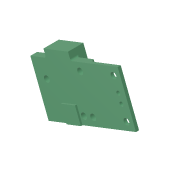
# Autodesk Inventor part: VWheelArmThickRIghtThinSwitchMount
Saved by Autodesk Inventor 2018 (Build 220112000, 112)
## iProperties
Created: 2018-12-14
Part Number: VWheelArmThickRIghtThinSwitchMount
Material: Generic
Document SubType Name: Modeling
Designer: ball
Density: 1 g/cm^3
Appearance: Default
Author: ball
Autodesk Inventor part; units mm, degrees
ref_plane "YZ Plane" through (0, 0, 0) normal (1, 0, 0) x (0, 1, 0)
ref_plane "XZ Plane" through (0, 0, 0) normal (0, 1, 0) x (-1, 0, 0)
ref_plane "XY Plane" through (0, 0, 0) normal (0, 0, 1) x (1, 0, 0)
sketch "Sketch1" plane through (0, 0, 0) normal (0, 0, 1) x (1, 0, 0)
  circle A0 centre (50.1681, 27.2834) radius 1.778 construction
  circle A1 centre (25.0574, 17.5233) radius 1.778 construction
  circle A2 centre (34.8176, -7.5874) radius 1.778 construction
  circle A3 centre (59.9282, 2.1728) radius 1.778 construction
  circle A4 centre (0, 0) radius 3.5 construction
  circle A5 centre (44.7061, 31.1467) radius 1.778 construction
  circle A6 centre (58.509, -4.3651) radius 1.778 construction
  circle A7 centre (26.4767, 24.0612) radius 1.778 construction
  circle A8 centre (40.2796, -11.4506) radius 1.778 construction
  line L0 (44.7061, 31.1467) -> (26.4767, 24.0612) construction
  line L1 (58.509, -4.3651) -> (40.2796, -11.4506) construction
  line L2 (168.5413, -268.1733) -> (30.5122, 86.945) construction
  circle A9 centre (-14.8554, 15.0432) radius 1.778 construction
  circle A10 centre (1.8062, -27.8234) radius 1.778 construction
  line L3 (67.1502, -1.0064) -> (1.3271, -26.5908)
  line L4 (53.3473, 34.5054) -> (-12.4758, 8.921)
  line L5 (-12.4758, 8.921) -> (1.3271, -26.5908)
  circle A11 centre (50.1681, 27.2834) radius 2.2479
  circle A12 centre (59.9282, 2.1728) radius 2.2479
  circle A13 centre (34.8176, -7.5874) radius 2.2479
  circle A14 centre (25.0574, 17.5233) radius 2.2479
  circle A15 centre (0, 0) radius 2.2479
  line L6 (53.3473, 34.5054) -> (67.1502, -1.0064)
  circle A16 centre (27.9489, -10.2481) radius 2.2479
  point P0 (51.2166, 33.6772)
  dimension "d0" = 4.4958
  dimension "d1" = 4.4958
  dimension "d2" = 4.4958
  dimension "d3" = 4.4958
  dimension "d4" = 4.4958
  dimension "d28" = 4.4958
  dimension "d29" = 7.366
  dimension "d30" = 5.5796
  dimension "d31" = 5.588
  constraints: 17 centre point, 14 end point, 5 coincident, 4 point on line, 28 other
  measures "d0" diameter of A11
  measures "d1" diameter of A12
  measures "d2" diameter of A13
  measures "d3" diameter of A14
  measures "d4" diameter of A15
  measures "d28" diameter of A16
  measures "d29" distance of A2.centre A16.centre
  measures "d30" distance from line of L3 A13.centre
  measures "d31" distance from line of L3 A16.centre
extrude "Extrusion1" add sketch "Sketch1" along normal blind 2.286 contours L3 L5 L4 L6 | A16
sketch "Sketch2" plane through (0, 0, 0) normal (0, 0, -1) x (-1, 0, 0)
  line L0 (12.4758, 8.921) -> (-1.3271, -26.5908) projected
  line L1 (12.4758, 8.921) -> (-1.3271, -26.5908)
  line L2 (-1.3271, -26.5908) -> (-43.9413, -10.0274)
  line L3 (-43.9413, -10.0274) -> (-30.1384, 25.4845)
  line L4 (-30.1384, 25.4845) -> (12.4758, 8.921)
  circle A0 centre (0, 0) radius 2.2479 projected
  circle A1 centre (-34.8176, -7.5874) radius 2.2479 projected
  circle A2 centre (-25.0574, 17.5233) radius 2.2479 projected
  dimension "d7" = 45.72
  constraints: 8 end point, 3 equal length, 1 perpendicular
  measures "d7" distance of L3.end L0.start
extrude "Extrusion2" add sketch "Sketch2" along normal blind 2.794
sketch "Sketch3" plane through (0, 0, -2.794) normal (0, 0, -1) x (-1, 0, 0)
  line L0 (-19.647, 16.2289) -> (-16.4172, 24.5387) construction
  line L1 (2.3869, 18.0201) -> (-1.1099, 9.0238) construction
  circle A0 centre (-5.0584, 13.1678) radius 1.1938 construction
  circle A1 centre (-13.9363, 16.6185) radius 1.1938 construction
  line L2 (-6.3321, 22.0903) -> (2.0251, 18.842) construction
  line L3 (-1.1099, 9.0238) -> (-19.647, 16.2289)
  line L4 (-19.647, 16.2289) -> (-15.9203, 25.8171)
  line L5 (-15.9203, 25.8171) -> (2.6169, 18.612)
  line L6 (2.6169, 18.612) -> (-1.1099, 9.0238)
  circle A2 centre (-5.0584, 13.1678) radius 1.1938
  circle A3 centre (-13.9363, 16.6185) radius 1.1938
  point P0 (0, 0)
  constraints: 14 end point, 4 centre point, 2 coincident, 2 concentric, 2 parallel, 1 perpendicular, 13 other
ref_plane "Work Plane1" through (-2.6408, 8.9775, -9.2647) normal (0, 0, 1) x (0.9320689, 0.3622811, 0)
extrude "Extrusion3" add sketch "Sketch3" along normal up to surface (6.4707 mm away)
sketch "Sketch4" plane through (0, 0, -2.794) normal (0, 0, 1) x (1, 0, 0)
  line L0 (-0.6385, 13.5219) -> (17.8987, 20.7271) projected
  line L1 (17.8987, 20.7271) -> (-0.6385, 13.5219)
  line L2 (-0.6385, 13.5219) -> (-2.6169, 18.612)
  line L3 (-2.6169, 18.612) -> (15.9203, 25.8171)
  line L4 (15.9203, 25.8171) -> (17.8987, 20.7271)
  point P0 (0, 0)
  constraints: 8 end point, 3 equal length, 1 perpendicular
extrude "Extrusion4" add sketch "Sketch4" along normal up to surface (5.08 mm away)
fillet "Fillet1" radius 3.175 1 edges at (37.0399, 7.7286, 0)
sketch "Sketch5" plane through (0, 0, 0) normal (0, 0, -1) x (-1, 0, 0)
  circle A0 centre (-50.1681, 27.2834) radius 2.2479 construction
  circle A1 centre (-59.9282, 2.1728) radius 2.2479 construction
  line L0 (-50.1681, 27.2834) -> (-59.9282, 2.1728) construction
  circle A2 centre (-53.8949, 17.6952) radius 1.524
  circle A3 centre (-56.1954, 11.7766) radius 1.524
  point P0 (0, 0)
  dimension "d15" = 3.048
  dimension "d16" = 3.048
  dimension "d17" = 6.35
  dimension "d18" = 10.287
  constraints: 2 centre point, 2 end point, 2 point on line
  measures "d15" diameter of A2
  measures "d16" diameter of A3
  measures "d17" distance of A3.centre A2.centre
  measures "d18" distance of A2.centre L0.start
extrude "Extrusion5" cut sketch "Sketch5" along normal through all both and the other way through all
fillet "Fillet2" radius 1.27 3 edges at (10.3785, 12.6263, -2.794) (18.7729, 18.478, -2.794) (0.2357, 11.2729, -2.794)
fillet "Fillet3" radius 1.27 4 edges at (17.8987, 20.7271, -3.429) (17.8987, 20.7271, -0.254) (-0.6385, 13.5219, -3.429) (-0.6385, 13.5219, -0.254)
sketch "Sketch7" plane through (0, 0, 2.286) normal (0, 0, 1) x (1, 0, 0)
  line L0 (16.1237, -20.8396) -> (11.7463, -9.5775)
  line L1 (1.3271, -26.5908) -> (67.1502, -1.0064) projected
  line L2 (11.7463, -9.5775) -> (22.4709, -5.409)
  line L3 (22.4709, -5.409) -> (26.8483, -16.6712)
  line L4 (-12.4758, 8.921) -> (1.3271, -26.5908) projected
  line L5 (16.1237, -20.8396) -> (26.8483, -16.6712)
  line L6 (43.9413, -10.0274) -> (1.3271, -26.5908) projected
  point P0 (0, 0)
  dimension "d24" = 15.875
  dimension "d25" = 27.3812
  constraints: 8 end point, 2 perpendicular, 1 collinear, 1 point on line
  measures "d24" distance between parallel lines of L4 L0
  measures "d25" distance between parallel lines of L3 L4
extrude "Extrusion6" add sketch "Sketch7" along normal blind 1.27
sketch "Sketch9" plane through (0, 0, -2.794) normal (0, 0, -1) x (-1, 0, 0)
  circle A0 centre (-27.9489, -10.2481) radius 2.2479
  line L0 (-43.9413, -10.0274) -> (-1.3271, -26.5908) projected
  circle A1 centre (-34.8176, -7.5874) radius 2.2479 projected
  point P0 (0, 0)
  dimension "d32" = 4.4958
  dimension "d33" = 5.588
  dimension "d34" = 7.366
  constraints: 1 centre point
  measures "d32" diameter of A0
  measures "d33" distance from line of L0 A0.centre
  measures "d34" distance of A0.centre A1.centre
extrude "Extrusion7" cut sketch "Sketch9" against normal through all contours A0
body "Solid1"
